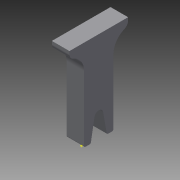
# Autodesk Inventor part: 27090914CameraMountB
Saved by Autodesk Inventor 2015 (Build 190159000, 159)
## iProperties
Created: 2013-05-28
Part Number: 27090914CameraMountB
Material: Generic
Document SubType Name: Modeling
Designer: Eric
Density: 1 g/cm^3
Appearance: Default
Author: Eric
Autodesk Inventor part; units mm, degrees
ref_plane "YZ Plane" through (0, 0, 0) normal (1, 0, 0) x (0, 1, 0)
ref_plane "XZ Plane" through (0, 0, 0) normal (0, 1, 0) x (-1, 0, 0)
ref_plane "XY Plane" through (0, 0, 0) normal (0, 0, 1) x (1, 0, 0)
sketch "Sketch1" plane through (0, 0, 0) normal (1, 0, 0) x (0, 1, 0)
  line L0 (-8.7654, 33.1522) -> (-8.7039, 33.1268)
  line L1 (8.7039, 33.1268) -> (8.7654, 33.1522)
  line L2 (-5, 27.5835) -> (-5, 5.5)
  line L3 (5, 27.5835) -> (5, 5.5)
  arc A0 (-5, 27.5835) -> (-8.7039, 33.1268) centre (-11, 27.5835) ccw
  arc A1 (8.7039, 33.1268) -> (5, 27.5835) centre (11, 27.5835) ccw
  arc A2 (1.4772, 12.2605) -> (-1.4772, 12.2605) centre (0, 12) ccw
  line L4 (0, 12) -> (0, 0) construction
  line L5 (-2.6846, 5.4132) -> (-1.4772, 12.2605)
  line L6 (2.6846, 5.4132) -> (1.4772, 12.2605)
  arc A3 (-2.9666, 3.8138) -> (-3.1376, 3.8439) centre (-3.0521, 3.8288) ccw
  arc A4 (3.1376, 3.8439) -> (2.9666, 3.8138) centre (3.0521, 3.8288) ccw
  line L7 (-10, 36) -> (10, 36)
  line L8 (-10, 36) -> (-10, 35)
  line L9 (10, 36) -> (10, 35)
  circle A5 centre (0, 0) radius 46 construction
  arc A6 (-10, 35) -> (-8.7654, 33.1522) centre (-8, 35) ccw
  arc A7 (8.7654, 33.1522) -> (10, 35) centre (8, 35) ccw
  line L10 (-4.5, 5) -> (-3.177, 5)
  line L11 (4.5, 5) -> (3.177, 5)
  arc A8 (-5, 5.5) -> (-4.5, 5) centre (-4.5, 5.5) ccw
  arc A9 (-3.177, 5) -> (-2.6846, 5.4132) centre (-3.177, 5.5) ccw
  arc A10 (2.6846, 5.4132) -> (3.177, 5) centre (3.177, 5.5) ccw
  arc A11 (4.5, 5) -> (5, 5.5) centre (4.5, 5.5) ccw
  point P0 (-5, 31.5926)
  point P1 (5, 31.5926)
  point P2 (-2.7574, 5)
  point P3 (-5, 5)
  point P4 (5, 5)
  point P5 (2.7574, 5)
  point P6 (-3.8385, 5)
  point P7 (3.8385, 5)
  dimension "d25" = 10
  dimension "d32" = 6
  dimension "d33" = 6
  dimension "d77" = 3
  dimension "d82" = 46
  dimension "d88" = 20
  dimension "d90" = 2
  dimension "d94" = 1
  dimension "d96" = 22.5
  dimension "d113" = 12
  dimension "d114" = 10
  dimension "d115" = 5
  dimension "d116" = 0.5
  dimension "d118" = 36
  constraints: 24 end point, 22 point on circle, 20 tangent, 15 point on line, 12 centre point, 6 coincident, 5 equal radius, 3 horizontal, 2 midpoint, 2 parallel, 2 vertical, 1 horizontal alignment, 1 perpendicular, 2 other
  measures "d25" distance between parallel lines of L2 L3
  measures "d32" radius of A0
  measures "d33" radius of A1
  measures "d77" diameter of A2
  measures "d82" radius of A5
  measures "d88" distance between parallel lines of L8 L9
  measures "d90" radius of A6
  measures "d94" distance from line of L7 A7.centre
  measures "d96" angle of L1 L7
  measures "d113" distance of L4.start point (0, 0)
  measures "d114" angle of L4 L6
  measures "d115" distance from line of point (0, 0) L10
  measures "d116" radius of A8
  measures "d118" distance from line of point (0, 0) L7
extrude "Extrusion7" add sketch "Sketch1" along normal blind 6
body "Solid7"
